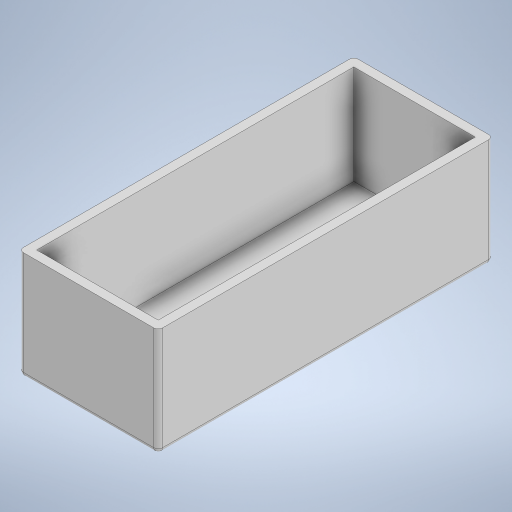
# Autodesk Inventor part: Battery Box Bottom
Saved by Autodesk Inventor 2024 (Build 280153000, 153)
## iProperties
Created: 2023-07-25
Part Number: Battery Box Bottom
Material: Generic
Document SubType Name: Modeling
Designer: techn
Density: 1 g/cm^3
Appearance: Default
Author: techn
## iProperties of the stored document Battery Box Bottom_3DPrint.ipt
Created: 2023-07-25
Part Number: Battery Box Bottom_3DPrint
Material: Generic
Document SubType Name: Modeling
Designer: techn
Density: 1 g/cm^3
Appearance: Default
Author: techn
Autodesk Inventor part; units mm, degrees
ref_plane "YZ Plane" through (0, 0, 0) normal (1, 0, 0) x (0, 1, 0)
ref_plane "XZ Plane" through (0, 0, 0) normal (0, 1, 0) x (-1, 0, 0)
ref_plane "XY Plane" through (0, 0, 0) normal (0, 0, 1) x (1, 0, 0)
sketch "Sketch3" plane through (0, 0, 0) normal (0, 1, 0) x (-1, 0, 0)
  line L0 (3.5626, 7.7011) -> (-78.4374, 7.7011)
  line L1 (-78.4374, -212.2989) -> (3.5626, -212.2989)
  line L2 (-84.4374, 13.7011) -> (9.5626, 13.7011)
  line L3 (9.5626, -212.2989) -> (3.5626, -212.2989)
  line L4 (-84.4374, -212.2989) -> (-78.4374, -212.2989)
  line L5 (-61.601, -206.2989) -> (-78.4374, -206.2989)
  line L6 (3.5626, -206.2989) -> (-61.601, -206.2989)
  line L7 (-84.4374, 13.7011) -> (-84.4374, -212.2989)
  line L8 (9.5626, 13.7011) -> (9.5626, -212.2989)
  line L9 (3.5626, -206.2989) -> (3.5626, 7.7011)
  line L10 (-78.4374, 7.7011) -> (-78.4374, -206.2989)
  point P0 (0, 0)
  dimension "d0" = 82
  dimension "d1" = 220
  constraints: 22 end point, 3 parallel, 3 vertical, 2 horizontal, 2 point on line, 1 collinear
  measures "d0" distance of L1.end L1.start
  measures "d1" distance of L1.start L0.end
extrude "Extrusion1" add sketch "Sketch3" along normal blind 6 contours L9 L6 L5 L10 L0 | L4 L7 L2 L8 L3 L1
sketch "Sketch4" plane through (0, 6, 0) normal (0, 1, 0) x (1, 0, 0)
  line L0 (-9.5626, 212.2989) -> (-9.5626, -13.7011) projected
  line L1 (-9.5626, -13.7011) -> (-3.5626, -13.7011)
  line L2 (-9.5626, -13.7011) -> (84.4374, -13.7011) projected
  line L3 (-3.5626, -13.7011) -> (-3.5626, -7.6991)
  line L4 (-3.5626, -7.6991) -> (78.4374, -7.6991)
  line L5 (78.4374, -7.6991) -> (78.4374, 206.3009)
  line L6 (78.4374, 206.3009) -> (-3.5626, 206.3009)
  line L7 (-3.5626, 206.3009) -> (-3.5626, -7.6991)
  line L8 (84.4374, 212.2989) -> (-9.5626, 212.2989) projected
  line L9 (-9.5626, -13.7011) -> (84.4374, -13.7011)
  line L10 (84.4374, -13.7011) -> (84.4374, 212.2989)
  line L11 (84.4374, 212.2989) -> (-9.5626, 212.2989)
  line L12 (-9.5626, 212.2989) -> (-9.5626, -13.7011)
  point P0 (0, 0)
  dimension "d9" = 6
  dimension "d10" = 82
  dimension "d11" = 214
  constraints: 20 end point, 4 parallel, 2 horizontal, 2 perpendicular, 1 point on line, 1 vertical
  measures "d9" distance of L0.end L1.end
  measures "d10" distance of L6.end L5.end
  measures "d11" distance of L5.end L4.end
extrude "Extrusion2" add sketch "Sketch4" along normal blind 67
fillet "Fillet1" radius 3 8 edges at (84.4374, 36.5, -212.2989) (-9.5626, 36.5, -212.2989) (-9.5626, 36.5, 13.7011) (84.4374, 36.5, 13.7011) (37.4374, 0, 13.7011) (84.4374, 0, -99.2989) (-9.5626, 0, -99.2989) (37.4374, 0, -212.2989)
body "Solid1"
